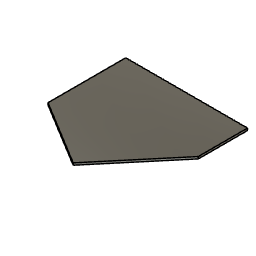
Base v2 (Autodesk Fusion 360 design; units mm, degrees)
Autodesk Fusion 360 part; units mm, degrees
sketch "Sketch1" plane through (0, 0, 0) normal (0, 0, 1) x (1, 0, 0) in component "Case "
  line L0 (0, 0) -> (117.5, 0)
  line L1 (117.5, 0) -> (117.5, -47.5)
  line L2 (117.5, -47.5) -> (62.4309, -113.1288)
  line L3 (0, 0) -> (0, -75)
  line L4 (0, -75) -> (62.4309, -113.1288)
  line L5 (0, -66.2119) -> (67.3065, -107.3183)
  line L6 (55.9577, -109.1753) -> (117.5, -35.8321)
  line L7 (0, -7.5) -> (117.5, -7.5)
  line L8 (110, 0) -> (110, -56.4382)
  line L9 (117.5, -47.5) -> (0, -47.5)
  dimension "d3" = 140
  dimension "d11" = 7.5
  dimension "d12" = 7.5
  dimension "d13" = 7.5
  dimension "d14" = 7.5
  dimension "d15" = 110
  dimension "d16" = 47.5
  dimension "d17" = 18.7119
  dimension "d18" = 75
  constraint coincident L0.start L3.start
  constraint horizontal L0
  constraint perpendicular L0 L1
  constraint coincident L3 L5.start
  constraint coincident L2 L5.end
  constraint parallel L4 L5
  constraint coincident L4 L6.start
  constraint coincident L1 L6.end
  constraint parallel L2 L6
  constraint coincident L3 L7.start
  constraint coincident L1 L7.end
  constraint perpendicular L1 L7
  constraint coincident L0 L8.start
  constraint perpendicular L0 L8
  constraint coincident L2 L8.end
  constraint coincident L3 L9.end
  constraint perpendicular L3 L9
  measures "d3" angle of L1 L2
  measures "d11" distance of L1 L8
  measures "d12" distance of L0 L7
  measures "d13" distance of L4 L5
  measures "d14" distance of L2 L6
  measures "d15" distance of L3 L8
  measures "d16" distance of L0 L9
  measures "d17" distance of L5.start L9.end
  measures "d18" distance of L3.end L0.start
extrude "Extrude1" add sketch "Sketch1" along normal blind 5
extrude "Extrude2" cut 1 faces at (59.1022, -70.4188, 5) along direction (0, 0, -1) blind 3
extrude "Extrude1'" [suppressed] in component "Case "
extrude "Extrude3" [suppressed] in component "Case "
sketch "Sketch2" plane through (0, 0, 0) normal (0, 0, 1) x (1, 0, 0) in component "Case "
  line L0 (0, 31.2783) -> (117.5, 31.2783)
  line L1 (117.5, 31.2783) -> (117.5, 78.7783)
  line L2 (117.5, 78.7783) -> (62.4311, 144.4069)
  line L3 (0, 31.2783) -> (0, 106.2783)
  line L4 (0, 106.2783) -> (62.4311, 144.4069)
  dimension "d23" = 117.5
  dimension "d24" = 47.5
  dimension "d25" = 85.672
  dimension "d29" = 75
  dimension "d31" = 140
  dimension "d32" = 73.1535
  constraint perpendicular L0 L1
  measures "d23" distance of L0.start L0.end
  measures "d24" distance of L0.end L1.end
  measures "d25" distance of L1.end L2.end
  measures "d29" distance of L0.start L3.end
  measures "d31" angle of L1 L2
  measures "d32" distance of L2.end L3.end
extrude "Extrude4" [suppressed] in component "Case "
extrude "Extrude5" [suppressed] in component "Case "
extrude "Extrude2'" [suppressed] in component "Case "
component "Case " placed x (1, 0, 0) y (0, 1, 0) z (0, 0, 1) at (0, 0, 0)
